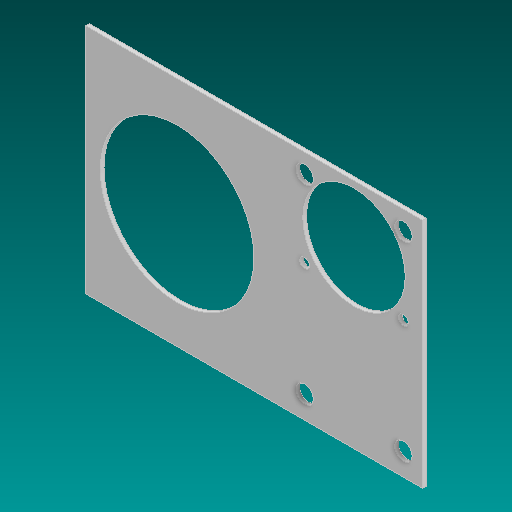
# Autodesk Inventor part: Part4
Saved by Autodesk Inventor 2020 (Build 240168000, 168)
## iProperties
Created: 2022-11-14
Part Number: Part4
Material: 一般
Document SubType Name: Modeling
Designer: Administrator
Density: 1 g/cm^3
Appearance: 既定
Author: Administrator
Autodesk Inventor part; units mm, degrees
ref_plane "YZ Plane" through (0, 0, 0) normal (1, 0, 0) x (0, 1, 0)
ref_plane "XZ Plane" through (0, 0, 0) normal (0, 1, 0) x (-1, 0, 0)
ref_plane "XY Plane" through (0, 0, 0) normal (0, 0, 1) x (1, 0, 0)
sketch "スケッチ1" plane through (0, 0, 0) normal (0, 0, 1) x (1, 0, 0)
  line L0 (14.5843, 13.35) -> (-14.5843, 13.35) projected
  line L1 (-14.5843, 13.35) -> (-16.35, 11.5843) projected
  line L2 (-16.35, 11.5843) -> (-16.35, -42.5843) projected
  line L3 (-16.35, -42.5843) -> (-14.5843, -44.35) projected
  line L4 (-14.5843, -44.35) -> (14.5843, -44.35) projected
  line L5 (14.5843, -44.35) -> (16.35, -42.5843) projected
  line L6 (16.35, -42.5843) -> (16.35, 11.5843) projected
  line L7 (16.35, 11.5843) -> (14.5843, 13.35) projected
  circle A0 centre (-13.5, 10.5) radius 2.4 projected
  circle A1 centre (13.5, -41.5) radius 2.4 projected
  circle A2 centre (-13.5, -41.5) radius 2.4 projected
  circle A3 centre (13.5, -10.5) radius 1.35 projected
  circle A4 centre (-13.5, -10.5) radius 1.35 projected
  circle A5 centre (13.5, 10.5) radius 2.4 projected
  circle A6 centre (0, 0) radius 13 projected
  line L8 (18.75, 15.75) -> (18.75, -47.6913) projected
  line L9 (-83.25, 15.75) -> (16.75, 15.75) projected
  line L10 (-73.341, 13.75) -> (-73.341, 3.75) projected
  line L11 (18.75, 15.75) -> (-73.341, 15.75)
  line L12 (-73.341, 15.75) -> (-73.341, -47.6913)
  line L13 (-73.341, -47.6913) -> (18.75, -47.6913)
  line L14 (18.75, -47.6913) -> (18.75, 15.75)
  line L15 (-52.6233, -21.6557) -> (-51.2333, -20.6912) projected
  arc A7 (-51.2333, -20.6912) -> (-53.5136, -17.4049) centre (-48.341, -16.25) ccw projected
  line L16 (-53.5136, -17.4049) -> (-54.9036, -18.3694) projected
  arc A8 (-54.9036, -18.3694) -> (-54.9539, -18.6477) centre (-54.7896, -18.5337) ccw projected
  line L17 (-54.9539, -18.6477) -> (-52.9016, -21.6054) projected
  arc A9 (-52.9016, -21.6054) -> (-52.6233, -21.6557) centre (-52.7373, -21.4914) ccw projected
  circle A10 centre (-48.341, -16.25) radius 19.7 projected
  circle A11 centre (0, 0) radius 14
  circle A12 centre (-48.341, -16.25) radius 21
  dimension "d0" = 28
  dimension "d1" = 42
  constraints: 8 end point, 2 centre point, 2 coincident, 2 parallel, 1 horizontal, 1 perpendicular
  measures "d0" diameter of A11
  measures "d1" diameter of A12
extrude "押し出し1" add sketch "スケッチ1" along normal blind 1 contours L7 L6 L5 L4 L3 L2 L1 L0 A11 | L8 L13 L12 L10 L9 L11
